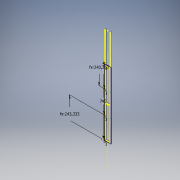
# Autodesk Inventor part: Makerbeam-Struktur
Saved by Autodesk Inventor 2018.2 (Build 222227000, 227)
## iProperties
Part Number: Makerbeam-Struktur
Material: Aluminium 6061
Document SubType Name: Modeling
Designer: makerstation
Density: 2.7 g/cm^3
Appearance: Aluminium - flach
Author: makerstation
Autodesk Inventor part; units mm, degrees
ref_plane "YZ Plane" through (0, 0, 0) normal (1, 0, 0) x (0, 1, 0)
ref_plane "XZ Plane" through (0, 0, 0) normal (0, 1, 0) x (-1, 0, 0)
ref_plane "XY Plane" through (0, 0, 0) normal (0, 0, 1) x (1, 0, 0)
sketch "Skizze2" plane through (0, 0, 0) normal (0, 1, 0) x (-1, 0, 0)
  line L0 (-35, 0) -> (-35, -1075)
  line L1 (-35, -1075) -> (35, -1075)
  line L2 (35, -1075) -> (35, 0)
  line L3 (-25, 0) -> (-25, -1075)
  line L4 (-25, -1065) -> (25, -1065)
  line L5 (25, -1075) -> (25, 0)
  line L6 (0, 28) -> (0, -210) construction
  line L7 (35, 0) -> (25, 0)
  line L8 (-25, 0) -> (-35, 0)
  line L9 (25, -350) -> (-25, -350)
  line L10 (-25, -350) -> (-25, -360)
  line L11 (-25, -360) -> (25, -360)
  line L12 (25, -360) -> (25, -350)
  line L13 (25, -705) -> (-25, -705)
  line L14 (-25, -705) -> (-25, -715)
  line L15 (-25, -715) -> (25, -715)
  line L16 (25, -715) -> (25, -705)
  point P0 (0, 0)
  dimension "d0" = 70
  dimension "d1" = 10
  dimension "laenge" = 1075
  dimension "d3" = 10
  dimension "d4" = 35
  dimension "d6" = 10
  dimension "d7" = 350
  dimension "d8" = 10
  dimension "d9" = 705
  constraints: 34 end point, 8 parallel, 8 point on line, 5 horizontal, 4 perpendicular, 1 vertical, 3 other
  measures "d0" distance of L0.end L1.end
  measures "d1" distance between parallel lines of L5 L2
  measures "laenge" distance of L0.start L0.end
  measures "d3" distance between parallel lines of L1 L4
  measures "d4" distance from line of L0 point (0, 0)
  measures "d6" distance of L10.end L9.end
  measures "d7" distance between parallel lines of L9 L7
  measures "d8" distance of L14.end L13.end
  measures "d9" distance between parallel lines of L7 L13
extrude "Extrusion1" add sketch "Skizze2" along normal blind 10 contours L8 L3 L1 L0 | L3 L4 L5 L1 | L9 L5 L11 L3 | L5 L7 L2 L1 | L3 L13 L5 L15
sketch "Skizze3" plane through (0, 0, 0) normal (0, -1, 0) x (1, 0, 0)
  line L0 (25, -715) -> (-25, -715) projected
  line L1 (25, -1065) -> (25, -715) projected
  line L2 (-25, -1065) -> (25, -1065) projected
  line L3 (-25, -715) -> (-25, -1065) projected
  line L4 (35, -1075) -> (-35, -1075) projected
  line L5 (35, 0) -> (35, -1075) projected
  line L6 (25, 0) -> (35, 0) projected
  line L7 (25, -350) -> (25, 0) projected
  line L8 (-25, -350) -> (25, -350) projected
  line L9 (-25, 0) -> (-25, -350) projected
  line L10 (-35, 0) -> (-25, 0) projected
  line L11 (-35, -1075) -> (-35, 0) projected
  line L12 (-25, -360) -> (-25, -705) projected
  line L13 (25, -360) -> (-25, -360) projected
  line L14 (25, -705) -> (25, -360) projected
  line L15 (-25, -705) -> (25, -705) projected
  line L16 (-35, -1075) -> (-35, 0) projected
  line L17 (35, -1075) -> (-35, -1075)
  line L18 (-35, -1075) -> (-35, -335)
  line L19 (-35, -335) -> (35, -335)
  line L20 (35, -335) -> (35, -1075)
  circle A0 centre (-30, -1070) radius 1.5
  circle A1 centre (-30, -340) radius 1.5
  line L21 (-30, -340) -> (-30, -1070) construction
  circle A2 centre (-30, -578.3333) radius 1.5
  circle A3 centre (-30, -831.6667) radius 1.5
  line L22 (0, -209.5174) -> (0, -1351.6434) construction
  circle A4 centre (30, -1070) radius 1.5
  circle A5 centre (30, -340) radius 1.5
  circle A6 centre (30, -578.3333) radius 1.5
  circle A7 centre (30, -831.6667) radius 1.5
  point P0 (0, 0)
  dimension "abdeckung" = 740
  dimension "d13" = 3
  dimension "d14" = 5
  dimension "d15" = 5
  dimension "d16" = 3
  dimension "d17" = 5
  dimension "d19" = 5
  dimension "d20" = 3
  dimension "d21" = 243.3333
  dimension "d22" = 3
  dimension "d23" = 243.3333
  constraints: 12 end point, 8 centre point, 4 symmetric about line, 3 point on line, 2 parallel, 1 horizontal, 1 perpendicular, 1 vertical, 4 other
  measures "abdeckung" distance of L17.end L18.end
  measures "d13" diameter of A0
  measures "d14" distance from line of L4 L21.end
  measures "d15" distance from line of L11 L21.end
  measures "d16" diameter of A1
  measures "d17" distance from line of L19 L21.start
  measures "d19" distance from line of L11 L21.start
  measures "d20" diameter of A2
  measures "d21" distance from line of L19 A2.centre
  measures "d22" diameter of A3
  measures "d23" distance from line of A3.centre L4
